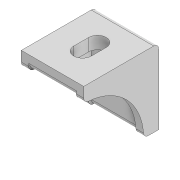
# Autodesk Inventor part: braket2
Saved by Autodesk Inventor 2020 (Build 240168000, 168)
## iProperties
Created: 2020-09-11
Part Number: braket2
Material: 일반
Document SubType Name: Modeling
Designer: 이호석
Mass: 7.05893 g
Surface Area: 41.1074 cm^2
Volume: 7.05893 cm^3
Density: 1 g/cm^3
Appearance: 기본값
Author: 이호석
Autodesk Inventor part; units mm, degrees
ref_plane "YZ Plane" through (0, 0, 0) normal (1, 0, 0) x (0, 1, 0)
ref_plane "XZ Plane" through (0, 0, 0) normal (0, 1, 0) x (-1, 0, 0)
ref_plane "XY Plane" through (0, 0, 0) normal (0, 0, 1) x (1, 0, 0)
sketch "스케치1" plane through (0, 0, 0) normal (0, 0, 1) x (1, 0, 0)
  line L0 (12.5, -15) -> (-12.5, -15)
  line L1 (-12.5, -15) -> (-12.5, 15)
  line L2 (-12.5, 15) -> (12.5, 15)
  line L3 (12.5, 15) -> (12.5, -15)
  line L4 (12.5, -15) -> (-12.5, 15) construction
  line L5 (-12.5, -15) -> (12.5, 15) construction
  point P0 (0, 0)
  dimension "d0" = 25
  dimension "d1" = 30
  constraints: 12 end point, 2 midpoint, 2 parallel, 1 horizontal, 1 perpendicular
  measures "d0" distance of L1.end L2.end
  measures "d1" distance of L0.end L1.end
extrude "돌출1" add sketch "스케치1" along normal blind 5
sketch "스케치2" plane through (0, 0, 5) normal (0, 0, 1) x (1, 0, 0)
  line L0 (12.5, 15) -> (-12.5, 15) projected
  line L1 (12.5, -15) -> (12.5, 15) projected
  line L2 (-12.5, 15) -> (12.5, 15)
  line L3 (12.5, 15) -> (12.5, 10)
  line L4 (12.5, 10) -> (-12.5, 10)
  line L5 (-12.5, 10) -> (-12.5, 15)
  point P0 (0, 0)
  dimension "d4" = 5
  constraints: 8 end point, 2 parallel, 1 horizontal, 1 perpendicular, 1 point on line
  measures "d4" distance of L2.end L3.end
extrude "돌출2" add sketch "스케치2" along normal blind 25
sketch "스케치3" plane through (0, 0, 5) normal (0, 0, 1) x (1, 0, 0)
  line L0 (0, -3) -> (0, 3) construction
  line L1 (3.5, -3) -> (3.5, 3)
  line L2 (-3.5, 3) -> (-3.5, -3)
  arc A0 (-3.5, -3) -> (3.5, -3) centre (0, -3) ccw
  arc A1 (3.5, 3) -> (-3.5, 3) centre (0, 3) ccw
  point P0 (0, 0)
  dimension "d7" = 3
  dimension "d8" = 7
  constraints: 8 end point, 4 point on circle, 4 tangent, 2 centre point, 1 midpoint, 1 parallel, 1 vertical
  measures "d7" distance of point (0, 0) L0.end
  measures "d8" diameter of A1
extrude "돌출3" cut sketch "스케치3" against normal through all
sketch "스케치4" plane through (-12.5, 10, 5) normal (0, -1, 0) x (1, 0, 0)
  line L0 (25, 0) -> (0, 0) projected
  line L1 (0, 0) -> (12.5, 0)
  line L2 (12.5, 7) -> (12.5, 13) construction
  line L3 (16, 7) -> (16, 13)
  line L4 (9, 13) -> (9, 7)
  arc A0 (9, 7) -> (16, 7) centre (12.5, 7) ccw
  arc A1 (16, 13) -> (9, 13) centre (12.5, 13) ccw
  point P0 (12.5, -5)
  dimension "d14" = 7
  constraints: 10 end point, 4 point on circle, 4 tangent, 2 centre point, 1 midpoint, 1 parallel, 1 vertical
  measures "d14" diameter of A1
extrude "돌출4" cut sketch "스케치4" against normal through all
sketch "스케치5" plane through (-12.5, -15, 0) normal (-1, 0, 0) x (0, 0, 1)
  line L0 (0, 30) -> (0, 0) projected
  line L1 (0, 0) -> (5, 0) projected
  line L2 (5, 25) -> (5, 0) projected
  line L3 (5, 25) -> (30, 25) projected
  line L4 (30, 30) -> (30, 25) projected
  line L5 (0, 30) -> (30, 30) projected
  line L6 (0, 0) -> (0, 30) projected
  line L7 (0, 30) -> (30, 30) projected
  line L8 (0, 0) -> (30, 0)
  line L9 (30, 0) -> (30, 30)
  line L10 (30, 30) -> (0, 30)
  line L11 (0, 30) -> (0, 0)
  line L12 (5, 0) -> (6, 0)
  line L13 (30, 25) -> (30, 24)
  line L14 (30, 24) -> (6, 0)
  circle A0 centre (30, 0) radius 24
  point P0 (0, 15)
  dimension "d17" = 1
  dimension "d18" = 1
  constraints: 14 end point, 2 parallel, 2 point on line, 1 coincident, 1 horizontal, 1 perpendicular, 3 other
  measures "d17" distance of L1.end L12.end
  measures "d18" distance of L3.end L13.end
extrude "돌출5" add sketch "스케치5" against normal blind 3 contours L2 L3 L9 A0 L8
sketch "스케치6" plane through (12.5, -15, 0) normal (1, 0, 0) x (0, 0, -1)
  line L0 (-30, 25) -> (-5, 25) projected
  line L1 (-30, 25) -> (-30, 24) projected
  arc A0 (-6, 0) -> (-30, 24) centre (-30, 0) ccw projected
  line L2 (-6, 0) -> (-5, 0) projected
  line L3 (-5, 25) -> (-5, 0) projected
  point P0 (0, 15)
extrude "돌출6" add sketch "스케치6" against normal blind 3
fillet "모깎기1" radius 2 8 edges at (-11, -15, 6) (0, -15, 5) (11, -15, 6) (0, 10, 30) (-11, 9, 30) (11, 9, 30) (0, 10, 5) (0, 15, 0)
